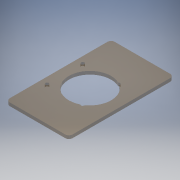
# Autodesk Inventor part: MotorMountDC
Saved by Autodesk Inventor 2019 (Build 230136000, 136)
## iProperties
Created: 2019-01-19
Part Number: MotorMountDC
Material: Polycarbonate, Smoke
Document SubType Name: Modeling
Designer: nxgam
Density: 1.2 g/cm^3
Appearance: Polycarbonate - Smoked
Author: nxgam
Autodesk Inventor part; units mm, degrees
ref_plane "YZ Plane" through (0, 0, 0) normal (1, 0, 0) x (0, 1, 0)
ref_plane "XZ Plane" through (0, 0, 0) normal (0, 1, 0) x (-1, 0, 0)
ref_plane "XY Plane" through (0, 0, 0) normal (0, 0, 1) x (1, 0, 0)
sketch "Sketch1" plane through (0, 0, 0) normal (0, 1, 0) x (-1, 0, 0)
  line L0 (-27.3558, 45.72) -> (27.3558, 45.72)
  line L1 (27.3558, 45.72) -> (27.3558, -45.72)
  line L2 (27.3558, -45.72) -> (-27.3558, -45.72)
  line L3 (-27.3558, -45.72) -> (-27.3558, 45.72)
  line L4 (-27.3558, 45.72) -> (27.3558, -45.72) construction
  line L5 (27.3558, 45.72) -> (-27.3558, -45.72) construction
  point P0 (0, 0)
  dimension "d0" = 54.7116
  dimension "d1" = 91.44
  constraints: 12 end point, 2 midpoint, 2 parallel, 1 horizontal, 1 perpendicular
  measures "d0" distance of L1.end L2.end
  measures "d1" distance of L0.end L1.end
extrude "Extrusion1" add sketch "Sketch1" along normal blind 2.794
fillet "Fillet1" radius 3.175 4 edges at (-27.3558, 1.397, 45.72) (27.3558, 1.397, 45.72) (27.3558, 1.397, -45.72) (-27.3558, 1.397, -45.72)
sketch "Sketch2" plane through (0, 2.794, 0) normal (0, 1, 0) x (1, 0, 0)
  circle A0 centre (-6.3442, 0) radius 6.223
  circle A1 centre (-12.7676, 7.75) radius 1.5
  circle A2 centre (14.0792, 7.75) radius 1.5
  circle A3 centre (0.6558, 15.5) radius 1.5
  circle A4 centre (0.6558, -15.5) radius 1.5
  circle A5 centre (14.0792, -7.75) radius 1.5
  circle A6 centre (-12.7676, -7.75) radius 1.5
  line L0 (-27.3558, -45.72) -> (-27.3558, 45.72)
  line L1 (-27.3558, 45.72) -> (27.3558, 45.72)
  line L2 (27.3558, 45.72) -> (27.3558, -45.72)
  line L3 (27.3558, -45.72) -> (-27.3558, -45.72)
  circle A7 centre (0, 0) radius 18.415
  dimension "d5" = 36.83
  constraints: 8 centre point, 8 end point, 2 horizontal, 2 vertical, 1 coincident, 18 other
  measures "d5" diameter of A7
extrude "Extrusion2" cut sketch "Sketch2" against normal blind 2.794 contours A0 | A1 | A2 | A3 | A4 | A5 | A6 | A7
sketch "Sketch3" plane through (0, 0, 0) normal (0, -1, 0) x (1, 0, 0)
  arc A0 (-39.5942, -30.48) -> (-36.5942, -30.48) centre (-38.0942, -30.48) ccw
  line L0 (-36.5942, -30.48) -> (-36.5942, -5.08)
  arc A1 (-36.5942, -5.08) -> (-39.5942, -5.08) centre (-38.0942, -5.08) ccw
  line L1 (-39.5942, -5.08) -> (-39.5942, -30.48)
  arc A2 (-39.5942, 5.08) -> (-36.5942, 5.08) centre (-38.0942, 5.08) ccw
  line L2 (-36.5942, 5.08) -> (-36.5942, 30.48)
  arc A3 (-36.5942, 30.48) -> (-39.5942, 30.48) centre (-38.0942, 30.48) ccw
  line L3 (-39.5942, 30.48) -> (-39.5942, 5.08)
  circle A4 centre (9.1558, -15.5) radius 1.5
  circle A5 centre (-21.8442, -15.5) radius 1.5
  circle A6 centre (9.1558, 15.5) radius 1.5
  circle A7 centre (-21.8442, 15.5) radius 1.5
  circle A8 centre (-6.3442, 0) radius 11
  line L4 (-10.7442, -50.8) -> (-20.9042, -50.8)
  line L5 (-20.9042, -50.8) -> (-20.9042, -45.72)
  line L6 (-20.9042, -45.72) -> (-31.0642, -45.72)
  line L7 (-31.0642, -45.72) -> (-31.0642, -50.8)
  line L8 (-31.0642, -50.8) -> (-41.2242, -50.8)
  line L9 (-41.2242, -50.8) -> (-41.2242, -45.72)
  line L10 (-41.2242, -45.72) -> (-46.3042, -45.72)
  line L11 (-46.3042, -45.72) -> (-46.3042, 45.72)
  line L12 (-46.3042, 45.72) -> (-41.2242, 45.72)
  line L13 (-41.2242, 45.72) -> (-41.2242, 50.8)
  line L14 (-41.2242, 50.8) -> (-31.0642, 50.8)
  line L15 (-31.0642, 50.8) -> (-31.0642, 45.72)
  line L16 (-31.0642, 45.72) -> (-20.9042, 45.72)
  line L17 (-20.9042, 45.72) -> (-20.9042, 50.8)
  line L18 (-20.9042, 50.8) -> (-10.7442, 50.8)
  line L19 (-10.7442, 50.8) -> (-10.7442, 45.72)
  line L20 (-10.7442, 45.72) -> (-0.5842, 45.72)
  line L21 (-0.5842, 45.72) -> (-0.5842, 50.8)
  line L22 (-0.5842, 50.8) -> (9.5758, 50.8)
  line L23 (9.5758, 50.8) -> (9.5758, 45.72)
  line L24 (9.5758, 45.72) -> (14.6558, 45.72)
  line L25 (14.6558, 45.72) -> (14.6558, -45.72)
  line L26 (14.6558, -45.72) -> (9.5758, -45.72)
  line L27 (9.5758, -45.72) -> (9.5758, -50.8)
  line L28 (9.5758, -50.8) -> (-0.5842, -50.8)
  line L29 (-0.5842, -50.8) -> (-0.5842, -45.72)
  line L30 (-0.5842, -45.72) -> (-10.7442, -45.72)
  line L31 (-10.7442, -45.72) -> (-10.7442, -50.8)
  point P0 (0, 0)
  constraints: 64 end point, 18 vertical, 14 horizontal, 9 centre point, 8 point on circle, 54 other
extrude "Extrusion3" cut sketch "Sketch3" against normal blind 2.794 contours A4 | A5 | A6 | A7
body "Solid1"
